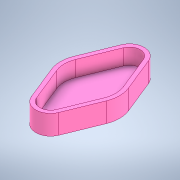
# Autodesk Inventor part: Diamond-Box
Saved by Autodesk Inventor 2022.4 (Build 264492000, 492)
## iProperties
Created: 2024-02-29
Part Number: Diamond-Box
Material: Generic
Document SubType Name: Modeling
Designer: t60147996
Density: 1 g/cm^3
Appearance: Pink
Author: t60147996
Autodesk Inventor part; units mm, degrees
ref_plane "YZ Plane" through (0, 0, 0) normal (1, 0, 0) x (0, 1, 0)
ref_plane "XZ Plane" through (0, 0, 0) normal (0, 1, 0) x (-1, 0, 0)
ref_plane "XY Plane" through (0, 0, 0) normal (0, 0, 1) x (1, 0, 0)
sketch "Sketch3" plane through (0, 0, 0) normal (0, 1, 0) x (-1, 0, 0)
  circle A0 centre (0, 0) radius 38.1
  circle A1 centre (0, -50.8) radius 19.05
  circle A2 centre (0, 50.8) radius 19.05
  line L0 (17.6598, 57.9438) -> (35.3196, 14.2875)
  line L1 (35.3196, -14.2875) -> (17.6598, -57.9438)
  line L2 (-17.6598, -57.9438) -> (-35.3196, -14.2875)
  line L3 (-17.6598, 57.9437) -> (-35.3196, 14.2875)
  constraints: 8 end point, 8 point on circle, 8 tangent, 3 centre point, 2 vertical alignment, 1 coincident
extrude "Extrusion2" add sketch "Sketch3" along normal blind 25.4
shell "Shell3" thickness 5.08 removed faces 1 at (-5.8866, 25.4, -28.8396)
body "Solid2"
